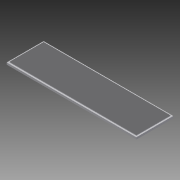
# Autodesk Inventor part: UNLHEP-14-01-P-011_Rubberstamp
Saved by Autodesk Inventor 2013 (Build 170138000, 138)
## iProperties
Created: 2014-01-22
Part Number: UNLHEP-14-01-P-011_Rubberstamp
Material: Allgemein
Document SubType Name: Modeling
Designer: Frank Meier
Density: 1 g/cm^3
Project: UNL Pixel Phase I
Author: Frank Meier
Autodesk Inventor part; units mm, degrees
ref_plane "YZ Plane" through (0, 0, 0) normal (1, 0, 0) x (0, 1, 0)
ref_plane "XZ Plane" through (0, 0, 0) normal (0, 1, 0) x (-1, 0, 0)
ref_plane "XY Plane" through (0, 0, 0) normal (0, 0, 1) x (1, 0, 0)
sketch "Skizze1" plane through (0, 0, 0) normal (0, 0, 1) x (1, 0, 0)
  line L0 (-32.5, -9.25) -> (32.5, -9.25)
  line L1 (32.5, -9.25) -> (32.5, 9.25)
  line L2 (32.5, 9.25) -> (-32.5, 9.25)
  line L3 (-32.5, 9.25) -> (-32.5, -9.25)
  line L4 (-32.5, -9.25) -> (32.5, 9.25) construction
  line L5 (32.5, -9.25) -> (-32.5, 9.25) construction
  point P0 (0, 0)
  dimension "d0" = 65
  dimension "d2" = 18.5
  constraints: 12 end point, 2 midpoint, 2 parallel, 1 horizontal, 1 perpendicular
  measures "d0" distance of L1.end L2.end
  measures "d2" distance of L2.end L0.start
extrude "Extrusion1" add sketch "Skizze1" along normal blind 1
sketch "Skizze2" plane through (0, 0, 1) normal (0, 0, 1) x (1, 0, 0)
  line L0 (32.5, 9.25) -> (-32.5, 9.25) projected
  line L1 (-32.5, 9.25) -> (-32.5, -9.25) projected
  line L2 (-31.8, -8.55) -> (31.8, -8.55)
  line L3 (31.8, -8.55) -> (31.8, 8.55)
  line L4 (31.8, 8.55) -> (-31.8, 8.55)
  line L5 (-31.8, 8.55) -> (-31.8, -8.55)
  line L6 (-31.8, 8.55) -> (31.9541, 8.55) construction
  line L7 (31.9541, 8.55) -> (31.9541, -8.7644) construction
  line L8 (31.9541, -8.7644) -> (-31.8, -8.7644) construction
  line L9 (-31.8, -8.7644) -> (-31.8, 8.55) construction
  point P0 (0, 0)
  dimension "d5" = 63.6
  dimension "d7" = 17.1
  dimension "d8" = 0.7
  dimension "d9" = 0.7
  constraints: 8 end point, 2 parallel, 1 horizontal, 1 perpendicular, 2 other
  measures "d5" distance of L3.end L4.end
  measures "d7" distance of L4.end L2.start
  measures "d8" distance between parallel lines of L1 L5
  measures "d9" distance between parallel lines of L0 L4
extrude "Extrusion2" add sketch "Skizze2" along normal blind 0.3
